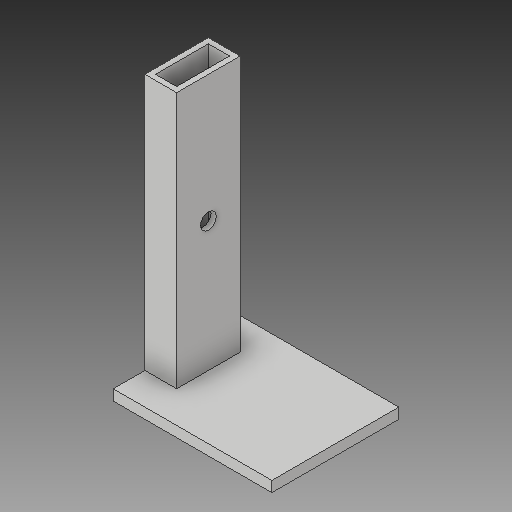
# Autodesk Inventor part: BasePostForSideOfRobot
Saved by Autodesk Inventor 2017 (Build 210142000, 142)
## iProperties
Created: 2016-02-12
Part Number: BasePostForSideOfRobot
Material: Generic
Document SubType Name: Modeling
Designer: steele
Density: 1 g/cm^3
Appearance: Default
Author: steele
Autodesk Inventor part; units mm, degrees
ref_plane "YZ Plane" through (0, 0, 0) normal (1, 0, 0) x (0, 1, 0)
ref_plane "XZ Plane" through (0, 0, 0) normal (0, 1, 0) x (-1, 0, 0)
ref_plane "XY Plane" through (0, 0, 0) normal (0, 0, 1) x (1, 0, 0)
sketch "Sketch1" plane through (0, 0, 0) normal (0, 1, 0) x (-1, 0, 0)
  line L0 (47.625, 38.1) -> (-47.625, 38.1)
  line L1 (-47.625, 38.1) -> (-47.625, -38.1)
  line L2 (-47.625, -38.1) -> (47.625, -38.1)
  line L3 (47.625, -38.1) -> (47.625, 38.1)
  line L4 (47.625, 38.1) -> (-47.625, -38.1) construction
  line L5 (-47.625, 38.1) -> (47.625, -38.1) construction
  point P0 (0, 0)
  dimension "d0" = 95.25
  dimension "d1" = 76.2
  constraints: 12 end point, 2 midpoint, 2 parallel, 1 horizontal, 1 perpendicular
  measures "d0" distance of L0.start L0.end
  measures "d1" distance of L2.end L0.start
extrude "Extrusion1" add sketch "Sketch1" against normal blind 6.35
sketch "Sketch4" plane through (0, 0, 0) normal (0, 1, 0) x (1, 0, 0)
  line L0 (-47.625, -19.05) -> (-28.575, -19.05)
  line L1 (-28.575, -19.05) -> (-28.575, 19.05)
  line L2 (-28.575, 19.05) -> (-47.625, 19.05)
  line L3 (-47.625, 19.05) -> (-47.625, -19.05)
  line L4 (-47.625, -19.05) -> (-28.575, 19.05) construction
  line L5 (-28.575, -19.05) -> (-47.625, 19.05) construction
  line L6 (-47.625, 38.1) -> (-47.625, -38.1) projected
  line L7 (-44.45, -15.875) -> (-31.75, -15.875)
  line L8 (-31.75, -15.875) -> (-31.75, 15.875)
  line L9 (-31.75, 15.875) -> (-44.45, 15.875)
  line L10 (-44.45, 15.875) -> (-44.45, -15.875)
  line L11 (-44.45, -15.875) -> (-31.75, 15.875) construction
  line L12 (-31.75, -15.875) -> (-44.45, 15.875) construction
  point P0 (0, 0)
  point P1 (-38.1, 0)
  dimension "d8" = 0
  dimension "d9" = 38.1
  dimension "d10" = 19.05
  dimension "d11" = 3.175
  dimension "d12" = 3.175
  constraints: 24 end point, 4 midpoint, 4 parallel, 2 horizontal, 2 perpendicular, 1 collinear
  measures "d8" vertical distance of point (0, 0) point (-38.1, 0)
  measures "d9" distance of L0.end L1.end
  measures "d10" distance of L0.start L0.end
  measures "d11" distance between parallel lines of L3 L10
  measures "d12" distance between parallel lines of L0 L7
extrude "Extrusion2" add sketch "Sketch4" along normal blind 153.924
sketch "Sketch5" plane through (-47.625, -6.35, -38.1) normal (-1, 0, 0) x (0, 0, 1)
  circle A0 centre (38.1, 84.074) radius 4.7625
  line L0 (19.05, 160.274) -> (57.15, 160.274) projected
  point P0 (38.1, 6.35)
  dimension "d15" = 9.525
  dimension "d16" = 76.2
  constraints: 1 centre point
  measures "d15" diameter of A0
  measures "d16" distance from line of A0.centre L0
extrude "Extrusion3" cut sketch "Sketch5" against normal through all
equation "\"d0\" = baseWidth"
equation "\"d1\" = baseLength"
equation "\"d2\" = baseThickness"
equation "\"d9\" = postLength"
equation "\"d10\" = postWidth"
equation "\"d11\" = postWallThickness"
equation "\"d12\" = postWallThickness"
equation "\"d13\" = postHeight"
equation "\"d15\" = postAxelDiam"
equation "\"d16\" = heightFromTopToAxelCenter"
equation "\"d17\" = postHeight"
equation "\"baseWidth\" = 95.25"
equation "\"baseLength\" = 76.2"
equation "\"baseThickness\" = 6.35"
equation "\"postWidth\" = 19.05"
equation "\"postLength\" = 38.1"
equation "\"postWallThickness\" = 3.175"
equation "\"postHeight\" = 153.924"
equation "\"postAxelDiam\" = 9.525"
equation "\"heightFromTopToAxelCenter\" = 76.2"
body "Solid1"
